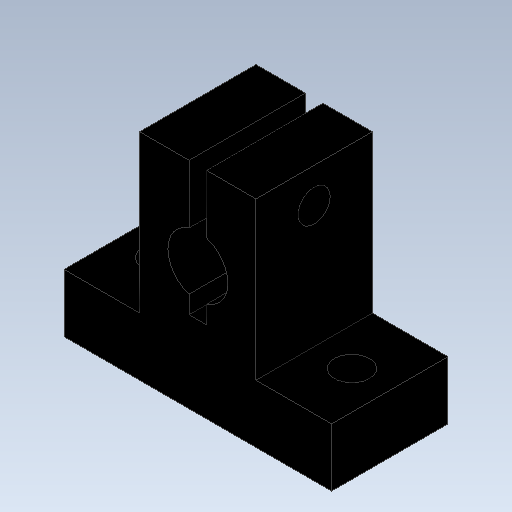
# Autodesk Inventor part: 0008-10-019 Suport Axa Y
Saved by Autodesk Inventor 2020 (Build 240168000, 168)
## iProperties
Created: 2021-02-27
Part Number: 0008-10-019 Suport Axa Y
Material: Generic
Document SubType Name: Modeling
Designer: Iulian Bors
Density: 1 g/cm^3
Appearance: Default
Description: Suport Axa
Mass: 16.5933 g
Surface Area: 65.9013 cm^2
Volume: 16.5933 cm^3
Author: Iulian Bors
Subject: 019
Autodesk Inventor part; units mm, degrees
ref_plane "YZ Plane" through (0, 0, 0) normal (1, 0, 0) x (0, 1, 0)
ref_plane "XZ Plane" through (0, 0, 0) normal (0, 1, 0) x (-1, 0, 0)
ref_plane "XY Plane" through (0, 0, 0) normal (0, 0, 1) x (1, 0, 0)
sketch "Sketch1" plane through (0, 0, 0) normal (0, 0, 1) x (1, 0, 0)
  line L0 (-23, 5) -> (23, 5)
  line L1 (23, 5) -> (23, -5)
  line L2 (23, -5) -> (-23, -5)
  line L3 (-23, -5) -> (-23, 5)
  line L4 (-10, 32) -> (10, 32)
  line L5 (10, 32) -> (10, 5)
  line L6 (10, 5) -> (-10, 5)
  line L7 (-10, 5) -> (-10, 32)
  circle A0 centre (0, 17) radius 5.15
  line L8 (-1.5, 32) -> (1.5, 32)
  line L9 (1.5, 32) -> (1.5, 9)
  line L10 (1.5, 9) -> (-1.5, 9)
  line L11 (-1.5, 9) -> (-1.5, 32)
  point P0 (0, 0)
  point P1 (-23, 0)
  point P2 (0, 5)
  point P3 (0, 32)
  point P4 (0, 32)
  point P5 (-1.5, 12.0733)
  point P6 (-1.5, 21.9267)
  point P7 (-1.5, 32)
  point P8 (-10, 5)
  point P9 (10, 5)
  point P10 (1.5, 32)
  point P11 (1.5, 21.9267)
  point P12 (1.5, 12.0733)
  dimension "d0" = 10
  dimension "d1" = 20
  dimension "d2" = 10.3
  dimension "d3" = 12
  dimension "d4" = 15
  dimension "d5" = 3
  dimension "d6" = 8
  dimension "d7" = 13
  constraints: 24 end point, 6 parallel, 4 midpoint, 3 horizontal, 3 perpendicular, 3 vertical alignment, 2 collinear, 1 centre point, 1 coincident, 1 horizontal alignment
  measures "d0" distance of L2.end L0.start
  measures "d1" distance of L4.start L4.end
  measures "d2" diameter of A0
  measures "d3" distance from line of L0 A0.centre
  measures "d4" distance from line of A0.centre L4
  measures "d5" distance between parallel lines of L11 L9
  measures "d6" distance from line of L10 A0.centre
  measures "d7" distance between parallel lines of L1 L5
extrude "Extrusion1" add sketch "Sketch1" along normal mid plane 20 contours L0 L1 L2 L3 | L7 L4 L11 A0 L10 L9 L5 L0
sketch "Sketch2" plane through (10, 5, 10) normal (0, 1, 0) x (1, 0, 0)
  line L0 (0, 20) -> (13, 20) projected
  line L1 (-33, 20) -> (-20, 20) projected
  line L2 (-33, 20) -> (-33, 0) projected
  line L3 (13, 20) -> (13, 0) projected
  point P0 (-10, 10)
  point P1 (-26.5, 10)
  point P2 (6.5, 10)
  point P3 (6.5, 20)
  point P4 (-26.5, 20)
  point P5 (-33, 10)
  point P6 (13, 10)
  constraints: 4 midpoint, 2 horizontal alignment, 2 vertical alignment
hole "Hole1" at (-16.5, 5, 0) at (16.5, 5, 0) direction (0, -1, 0) diameter 6 end through all
sketch "Sketch3" plane through (10, 5, 10) normal (1, 0, 0) x (0, 0, -1)
  line L0 (20, 27) -> (0, 27) projected
  circle A0 centre (10, 21) radius 2.75
  line L1 (20, 27) -> (0, 27) projected
  line L2 (0, 27) -> (8, 27)
  line L3 (8, 27) -> (8, 0)
  line L4 (8, 0) -> (0, 0)
  line L5 (0, 0) -> (0, 27)
  line L6 (20, 0) -> (0, 0) projected
  line L7 (12, 27) -> (20, 27)
  line L8 (20, 27) -> (20, 0)
  line L9 (20, 0) -> (12, 0)
  line L10 (12, 0) -> (12, 27)
  line L11 (20, 27) -> (20, 0) projected
  point P0 (10, -5)
  point P1 (10, 27)
  point P2 (12, 0)
  dimension "d17" = 6
  dimension "d18" = 5.5
  dimension "d19" = 8
  dimension "d21" = 8
  constraints: 16 end point, 4 collinear, 4 parallel, 2 horizontal, 2 perpendicular, 1 centre point, 1 coincident, 1 midpoint, 1 vertical alignment
  measures "d17" distance from line of point (10, 21) L0
  measures "d18" diameter of A0
  measures "d19" distance between parallel lines of L3 L5
  measures "d21" distance between parallel lines of L8 L10
extrude "Extrusion2" cut sketch "Sketch3" against normal through all contours L10 A0 L3 | A0 L10 | L3 A0
equation "\"d21\" = d19"
body "Solid1"
